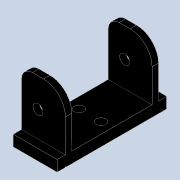
# Autodesk Inventor part: X Axis Drag Chain Mount Statonary Bolted
Saved by Autodesk Inventor 2022 (Build 260153000, 153)
## iProperties
Created: 2021-10-30
Part Number: X Axis Drag Chain Mount Statonary Bolted
Material: Generic
Document SubType Name: Modeling
Designer: Coy
Density: 1 g/cm^3
Appearance: Anodized - Black
Author: Coy
Autodesk Inventor part; units mm, degrees
ref_plane "YZ Plane" through (0, 0, 0) normal (1, 0, 0) x (0, 1, 0)
ref_plane "XZ Plane" through (0, 0, 0) normal (0, 1, 0) x (-1, 0, 0)
ref_plane "XY Plane" through (0, 0, 0) normal (0, 0, 1) x (1, 0, 0)
sketch "Sketch1" plane through (0, 0, 0) normal (0, 1, 0) x (-1, 0, 0)
  line L0 (0, 0) -> (24, 0)
  line L1 (24, 0) -> (24, 60)
  line L2 (24, 60) -> (0, 60)
  line L3 (0, 60) -> (0, 0)
  line L4 (24, 30) -> (0, 30) construction
  circle A0 centre (18, 30) radius 2.6
  circle A1 centre (6, 30) radius 2.6
  dimension "d0" = 24
  dimension "d1" = 60
  dimension "d2" = 5.2
  dimension "d3" = 5.2
  dimension "d4" = 6
  dimension "d5" = 6
  dimension "d6" = 12
  constraints: 10 end point, 2 centre point, 2 midpoint, 2 parallel, 2 point on line, 1 horizontal, 1 perpendicular
  measures "d0" distance of L2.end L1.end
  measures "d1" distance of L1.end L0.end
  measures "d2" diameter of A0
  measures "d3" diameter of A1
  measures "d4" distance from line of L1 A0.centre
  measures "d5" distance from line of L3 A1.centre
  measures "d6" distance of A1.centre A0.centre
extrude "Extrusion1" add sketch "Sketch1" along normal blind 6
sketch "Sketch2" plane through (0, 6, 0) normal (0, 1, 0) x (1, 0, 0)
  line L0 (-24, 0) -> (-24, -60) projected
  line L1 (-24, -4.5) -> (0, -4.5)
  line L2 (0, -4.5) -> (0, -8)
  line L3 (0, -8) -> (-24, -8)
  line L4 (-24, -8) -> (-24, -4.5)
  line L5 (-24, -55.5) -> (0, -55.5)
  line L6 (0, -55.5) -> (0, -52)
  line L7 (0, -52) -> (-24, -52)
  line L8 (-24, -52) -> (-24, -55.5)
  line L9 (0, 0) -> (-24, 0) projected
  dimension "d9" = 24
  dimension "d10" = 24
  dimension "d12" = 51
  dimension "d13" = 3.5
  dimension "d14" = 3.5
  dimension "d15" = 4.5
  constraints: 16 end point, 4 parallel, 2 horizontal, 2 perpendicular, 2 point on line
  measures "d9" distance of L2.end L3.end
  measures "d10" distance of L7.end L6.end
  measures "d12" distance between parallel lines of L1 L5
  measures "d13" distance between parallel lines of L1 L3
  measures "d14" distance between parallel lines of L5 L7
  measures "d15" distance between parallel lines of L9 L1
extrude "Extrusion2" add sketch "Sketch2" along normal blind 30
sketch "Sketch3" plane through (-24, 6, 55.5) normal (0, 0, 1) x (1, 0, 0)
  point P0 (24, -6)
sketch "Sketch4" plane through (-24, 6, 55.5) normal (0, 0, 1) x (1, 0, 0)
  circle A0 centre (9, 14) radius 2.75
  line L0 (0, 0) -> (24, 0) projected
  line L1 (0, 0) -> (0, 30) projected
  point P0 (24, -6)
  dimension "d18" = 5.5
  dimension "d19" = 14
  dimension "d20" = 9
  constraints: 1 centre point
  measures "d18" diameter of A0
  measures "d19" distance from line of L0 A0.centre
  measures "d20" distance from line of L1 A0.centre
extrude "Extrusion3" cut sketch "Sketch4" against normal through all
fillet "Fillet1" radius 12 2 edges at (0, 36, 53.75) (0, 36, 6.25)
fillet "Fillet2" radius 6 2 edges at (-24, 36, 53.75) (-24, 36, 6.25)
equation "\"d5\" = d4"
equation "\"d14\" = d13"
body "Solid1"
